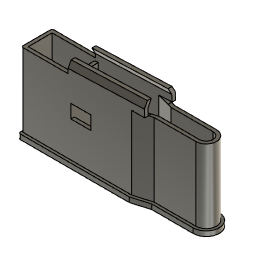
desert_tech_srs_magazine (Autodesk Fusion 360 design; units mm, degrees)
Autodesk Fusion 360 part; units mm, degrees
sketch "Sketch1" plane through (0, 0, 0) normal (0, 0, 1) x (1, 0, 0)
  line L0 (1.5, 0) -> (63.5, 0)
  line L1 (104, -3.9438) -> (104, 21.6938) construction
  line L2 (63.5, 17.75) -> (1.5, 17.75)
  line L3 (0, 16.25) -> (0, 1.5)
  line L4 (63.5, 17.75) -> (73.5, 14.8)
  line L5 (73.5, 14.8) -> (97.5, 14.8)
  line L6 (0, 8.875) -> (104, 8.875) construction
  arc A0 (103.425, 8.875) -> (97.5, 14.8) centre (97.5, 8.875) ccw
  line L7 (63.5, 0) -> (73.5, 2.95)
  line L8 (73.5, 2.95) -> (97.5, 2.95)
  arc A1 (97.5, 2.95) -> (103.425, 8.875) centre (97.5, 8.875) ccw
  line L9 (26.5, 15.75) -> (26.5, 11.375)
  line L10 (28.5, 11.375) -> (28.5, 15.75)
  line L11 (26.5, 2) -> (26.5, 6.375)
  line L12 (28.5, 6.375) -> (28.5, 2)
  arc A2 (101.425, 8.8708) -> (97.5, 12.8) centre (97.5, 8.875) ccw
  line L13 (73.3211, 12.8) -> (97.5, 12.8)
  line L14 (63.3211, 15.75) -> (73.3211, 12.8)
  line L15 (2, 15.75) -> (2, 2)
  line L16 (64.6249, 2) -> (74.6249, 4.95)
  line L17 (74.6249, 4.95) -> (97.5, 4.95)
  arc A3 (97.5, 4.95) -> (101.425, 8.8708) centre (97.5, 8.875) ccw
  line L18 (63.3211, 15.75) -> (28.5, 15.75)
  line L19 (26.5, 15.75) -> (2, 15.75)
  line L20 (2, 2) -> (26.5, 2)
  line L21 (28.5, 2) -> (64.6249, 2)
  line L22 (0, 1.5) -> (0, 0)
  line L23 (0, 0) -> (1.5, 0)
  line L24 (0, 16.25) -> (0, 17.75)
  line L25 (0, 17.75) -> (1.5, 17.75)
  line L26 (26.5, 11.375) -> (26.5, 6.375)
  line L27 (28.5, 11.375) -> (28.5, 6.375)
  point P0 (0, 17.75)
  dimension "d2" = 17.75
  dimension "d3" = 63.5
  dimension "d4" = 24
  dimension "d5" = 6.5
  dimension "d6" = 11.85
  dimension "d9" = 104
  dimension "d21" = 75.5
  dimension "d23" = 2
  dimension "d40" = 2
  dimension "d41" = 2
  dimension "d42" = 2
  constraint horizontal L0
  constraint vertical L1
  constraint horizontal L2
  constraint vertical L3
  constraint coincident L22.end L23.start
  constraint parallel L2 L5
  constraint midpoint L1 L6.end
  constraint coincident L6 A0.centre
  constraint tangent L5 A0
  constraint coincident L6 A0.start
  constraint symmetric L2.start L6 L0.end
  constraint symmetric L4.end L6 L7.end
  constraint symmetric L5.end L6 L8.end
  constraint symmetric L6 A0 A1
  constraint symmetric L6 A0.start A1.end
  constraint coincident L3 L6.start
  constraint coincident P0 L2
  constraint coincident P0 L3
  constraint coincident L22.end L3
  constraint coincident L22.end L0
  constraint symmetric L0 L2 L6
  constraint vertical L9
  constraint vertical L10
  constraint symmetric L6 L10.end L12.end
  constraint symmetric L6 L9.start L11.start
  constraint symmetric L6 L9.end L11.end
  constraint symmetric L6 L10.start L12.start
  constraint concentric A0 A2
  constraint parallel L5 L13
  constraint parallel L4 L14
  constraint parallel L2 L18
  constraint parallel L3 L15
  constraint parallel L0 L20
  constraint parallel L7 L16
  constraint parallel L8 L17
  constraint concentric A1 A3
  constraint tangent A2 A3
  constraint tangent A2 L13
  constraint tangent L17 A3
  constraint collinear L18 L19
  constraint collinear L20 L21
  constraint coincident P0 L24.end
  constraint parallel L12 L27
  measures "d2" distance of L22.end P0
  measures "d3" distance of L3 L2.start
  measures "d4" distance of L4.end L5.end
  measures "d5" distance of L1 L5.end
  measures "d6" diameter of A0
  measures "d9" distance of L1 L3
  measures "d21" distance of L1 L10
  measures "d23" distance of L9 L10
  measures "d40" distance of L2 L19
  measures "d41" distance of L5 L13
  measures "d42" distance of L3 L15
extrude "Extrude1" add sketch "Sketch1" along normal blind 45
sketch "Sketch2" plane through (0, 0, 0) normal (0, -1, 0) x (1, 0, 0)
  line L0 (0, 0) -> (63.5, 0)
  line L1 (63.5, 0) -> (63.5, 45)
  line L2 (63.5, 45) -> (0, 45)
  line L3 (28.5, 31) -> (40, 31)
  line L4 (40, 31) -> (40, 23.25)
  line L5 (40, 23.25) -> (28.5, 23.25)
  line L6 (28.5, 23.25) -> (28.5, 31)
  line L7 (0, 45) -> (0, 0)
  line L8 (0, 0) -> (0, 45)
  dimension "d25" = 7.75
  dimension "d26" = 11.5
  dimension "d28" = 14
  dimension "d36" = 28.5
  constraint horizontal L3
  constraint vertical L4
  constraint horizontal L5
  constraint vertical L6
  measures "d25" distance of L3 L5
  measures "d26" distance of L4 L6
  measures "d28" distance of L2 L3
  measures "d36" distance of L6 L8
extrude "Extrude2" cut sketch "Sketch2" against normal up to surface (2 mm away) contours L3 L4 L5 L6
sketch "Sketch4" plane through (0, 0, 0) normal (0, 1, 0) x (1, 0, 0)
  line L0 (0, -50) -> (70.7206, -52.6) construction
  line L1 (71, -45) -> (0, -45) construction
  line L2 (63.5, 0) -> (63.5, -45)
  line L3 (70.7206, -52.6) -> (71, -45)
  line L4 (63.5, -45) -> (73.5, -45)
  line L5 (0, -50) -> (0, -45) construction
  line L6 (26.9, -45) -> (26.9, -50.989)
  line L7 (0, 0) -> (0, -45)
  line L8 (26.9, -50.989) -> (70.7206, -52.6)
  line L9 (26.9, -45) -> (71, -45)
  point P0 (0, -45)
  dimension "d37" = 7.6
  dimension "d38" = 7.5
  dimension "d47" = 5
  dimension "d50" = 26.9
  constraint perpendicular L0 L3
  constraint coincident P0 L1.end
  constraint coincident L1.start L4
  constraint perpendicular L1 L5
  constraint coincident L1 L6.start
  constraint coincident L0 L6.end
  constraint perpendicular L1 L6
  measures "d37" distance of L0.end L1
  measures "d38" distance of L2.end L1.start
  measures "d47" distance of L1 L0.start
  measures "d50" distance of L6 L7
extrude "Extrude3" add sketch "Sketch4" along normal up to surface (17.75 mm away)
sketch "Sketch5" plane through (72.5563, 0, 2.6675) normal (0.999325, 0, 0.03674) x (0, 1, 0)
  line L0 (17.75, 42.3611) -> (17.75, 49.9662)
  line L1 (0, 49.9662) -> (0, 42.3611)
  line L2 (2.2125, 42.3611) -> (3.8807, 42.3611)
  line L3 (8.875, 53.3078) -> (8.875, 25.9939) construction
  line L4 (2, 46.1075) -> (2, 42.3611)
  line L5 (0, 42.3611) -> (2.2125, 42.3611)
  line L6 (2.2125, 42.3611) -> (12.4801, 42.3611)
  line L7 (12.4801, 42.3611) -> (12.4801, 42.3609)
  line L8 (12.4801, 42.3609) -> (15.5375, 42.3609)
  line L9 (15.5375, 42.3609) -> (12.4801, 42.361)
  line L10 (12.4801, 49.9662) -> (0, 49.9662)
  line L11 (0, 49.9662) -> (0, 42.3611)
  line L12 (2, 46.1075) -> (4.075, 49.9662)
  line L13 (0, 46.6112) -> (1.8042, 49.9662)
  line L14 (15.75, 46.1075) -> (13.675, 49.9662)
  line L15 (17.75, 46.6112) -> (15.9458, 49.9662)
  line L16 (15.75, 46.1075) -> (15.75, 42.3611)
  line L17 (17.75, 49.9662) -> (0, 49.9662)
  line L18 (0, 42.3611) -> (2.2125, 42.3611)
  line L19 (3.8807, 42.3611) -> (13.4847, 42.3611)
  line L20 (13.4847, 42.3611) -> (15.5375, 42.3611)
  line L21 (15.5375, 42.3611) -> (17.75, 42.3611)
  dimension "d49" = 2
  dimension "d51" = 2
  dimension "d56" = 9.6
  constraint vertical L3
  constraint symmetric L0 L1 L3
  constraint coincident L10 L12.end
  constraint coincident L11 L13.start
  constraint coincident L10 L13.end
  constraint parallel L12 L13
  constraint parallel L1 L4
  constraint symmetric L3 L4.end L16.end
  constraint symmetric L3 L4.start L14.start
  constraint symmetric L3 L12.end L14.end
  constraint symmetric L3 L13.start L15.start
  constraint symmetric L3 L13.end L15.end
  constraint parallel L2 L6
  constraint parallel L1 L11
  constraint collinear L6 L19
  measures "d49" distance of L12 L13
  measures "d51" distance of L4 L11
  measures "d56" distance of L12.end L14.end
extrude "Extrude4" cut sketch "Sketch5" along normal up to surface contours L0 L15 L17 | L2 L4 L5 L6 L8 L9 L10 L12 L14 L16 L17 L18 L19 L20 L21 | L1 L10 L11 L13 L17 end surface through (26.5, 2, 0) normal (-1, 0, 0) offset 0
sketch "Sketch8" plane through (0, 0, 0) normal (0, 0, -1) x (1, 0, 0)
  line L0 (63.3211, -15.75) -> (28.5, -15.75)
  line L1 (28.5, -15.75) -> (28.5, -2)
  line L2 (28.5, -2) -> (64.6249, -2)
  line L3 (64.6249, -2) -> (74.6249, -4.95)
  line L4 (74.6249, -4.95) -> (97.5, -4.95)
  arc A0 (97.5, -12.8) -> (97.5, -4.95) centre (97.5, -8.875) ccw
  line L5 (97.5, -12.8) -> (73.3211, -12.8)
  line L6 (73.3211, -12.8) -> (63.3211, -15.75)
  line L7 (2, -15.75) -> (2, -2)
  line L8 (2, -2) -> (26.5, -2)
  line L9 (26.5, -2) -> (26.5, -15.75)
  line L10 (0, 0) -> (0, -17.75)
  line L11 (0, -17.75) -> (63.5, -17.75)
  line L12 (63.5, -17.75) -> (73.5, -14.8)
  line L13 (73.5, -14.8) -> (97.5, -14.8)
  arc A1 (97.5, -14.8) -> (97.5, -2.95) centre (97.5, -8.875) ccw
  line L14 (97.5, -2.95) -> (73.5, -2.95)
  line L15 (73.5, -2.95) -> (63.5, 0)
  line L16 (63.5, 0) -> (0, 0)
  line L17 (0, -19.35) -> (63.7311, -19.35)
  line L18 (63.7311, -19.35) -> (73.7311, -16.4)
  line L19 (73.7311, -16.4) -> (97.5, -16.4)
  arc A2 (97.5, -16.4) -> (97.5, -1.35) centre (97.5, -8.875) ccw
  line L20 (97.5, -1.35) -> (73.7311, -1.35)
  line L21 (73.7311, -1.35) -> (63.7311, 1.6)
  line L22 (63.7311, 1.6) -> (0, 1.6)
  line L23 (0, -17.75) -> (63.5, -17.75)
  line L24 (63.5, -17.75) -> (73.5, -14.8)
  line L25 (73.5, -14.8) -> (97.5, -14.8)
  arc A3 (97.5, -14.8) -> (97.5, -2.95) centre (97.5, -8.875) ccw
  line L26 (97.5, -2.95) -> (73.5, -2.95)
  line L27 (73.5, -2.95) -> (63.5, 0)
  line L28 (63.5, 0) -> (0, 0)
  line L29 (0, 0) -> (0, -17.75)
  line L30 (0, 0) -> (0, 1.6)
  line L31 (0, -17.75) -> (0, -19.35)
  line L32 (26.5, -15.75) -> (2, -15.75)
  dimension "d53" = 0
  constraint coincident L10.start L16.end
  constraint perpendicular L22 L30
  constraint perpendicular L17 L31
  constraint parallel L11 L17
  constraint parallel L12 L18
  constraint parallel L13 L19
  constraint concentric A1 A2
  constraint parallel L14 L20
  constraint parallel L15 L21
  constraint parallel L16 L22
  constraint tangent A2 L20
  constraint tangent L19 A2
  measures "d53" distance of L11
extrude "Extrude5" add sketch "Sketch8" against normal blind 2.8 contours L11 L12 L13 A1 L14 L15 L16 L17 L18 L19 A2 L20 L21 L22 L23 L24 L25 A3 L26 L27 L28 L30 L31
fillet "Fillet1" radius 1 4 edges at (0, 0, 23.9) (0, 17.75, 23.9) (0, -1.6, 1.4) (0, 19.35, 1.4)
